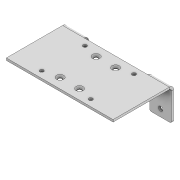
# Autodesk Inventor part: CCM_Mount_F
Saved by Autodesk Inventor 2020 (Build 240168000, 168)
## iProperties
Created: 2021-07-12
Part Number: CCM_Mount_F
Material: 一般
Document SubType Name: Sheet Metal
Designer: magnarecta
Density: 1 g/cm^3
Appearance: 既定
Sheet Metal Rule: Default
Author: magnarecta
Autodesk Inventor part; units mm, degrees
ref_plane "YZ Plane" through (0, 0, 0) normal (1, 0, 0) x (0, 1, 0)
ref_plane "XZ Plane" through (0, 0, 0) normal (0, 1, 0) x (-1, 0, 0)
ref_plane "XY Plane" through (0, 0, 0) normal (0, 0, 1) x (1, 0, 0)
sketch "スケッチ1" plane through (0, 0, 0) normal (0, 1, 0) x (-1, 0, 0)
  line L0 (-40, -39) -> (40, -39)
  line L1 (40, -39) -> (40, 39)
  line L2 (40, 39) -> (-40, 39)
  line L3 (-40, 39) -> (-40, -39)
  line L4 (-40, -39) -> (40, 39) construction
  line L5 (40, -39) -> (-40, 39) construction
  point P0 (0, 0)
  dimension "d0" = 80
  dimension "d1" = 78
  constraints: 12 end point, 2 midpoint, 2 parallel, 1 horizontal, 1 perpendicular
  measures "d0" distance of L0.start L0.end
  measures "d1" distance of L0.end L1.end
extrude "押し出し1" add sketch "スケッチ1" along normal blind 3
sketch "スケッチ2" plane through (0, 3, 0) normal (0, 1, 0) x (1, 0, 0)
  line L0 (34, 30) -> (-34, 30)
  line L1 (-34, 30) -> (-34, -30)
  line L2 (-34, -30) -> (34, -30)
  line L3 (34, -30) -> (34, 30)
  line L4 (34, 30) -> (-34, -30) construction
  line L5 (-34, 30) -> (34, -30) construction
  point P0 (0, 0)
  dimension "d4" = 68
  dimension "d5" = 60
  constraints: 12 end point, 2 midpoint, 2 parallel, 1 horizontal, 1 perpendicular
  measures "d4" distance of L2.end L1.end
  measures "d5" distance of L1.end L0.end
hole "穴1" at (-34, 3, 30) at (34, 3, 30) at (34, 3, -30) at (-34, 3, -30) direction (0, -1, 0) diameter 5.2 depth 8 tip angle 118
sketch "スケッチ3" plane through (0, 3, 0) normal (0, 1, 0) x (1, 0, 0)
  line L0 (13.5, 25) -> (-13.5, 25)
  line L1 (-13.5, 25) -> (-13.5, -25)
  line L2 (-13.5, -25) -> (13.5, -25)
  line L3 (13.5, -25) -> (13.5, 25)
  line L4 (13.5, 25) -> (-13.5, -25) construction
  line L5 (-13.5, 25) -> (13.5, -25) construction
  point P0 (0, 0)
  dimension "d13" = 27
  dimension "d14" = 50
  constraints: 12 end point, 4 coincident, 2 midpoint, 2 parallel, 1 horizontal, 1 perpendicular
  measures "d13" distance of L0.start L0.end
  measures "d14" distance of L0.end L1.end
hole "穴2" at (-13.5, 3, 25) at (13.5, 3, 25) at (13.5, 3, -25) at (-13.5, 3, -25) direction (0, -1, 0) diameter 5.3 depth 8 tip angle 118 countersink diameter 10 countersink angle 90
sketch "スケッチ5" plane through (0, 0, 0) normal (0, -1, 0) x (1, 0, 0)
  line L0 (74, 39) -> (-74, 39)
  line L1 (-74, 39) -> (-74, -39)
  line L2 (-74, -39) -> (74, -39)
  line L3 (74, -39) -> (74, 39)
  circle A0 centre (13.5, -25) radius 2.65 projected
  circle A1 centre (34, -30) radius 2.6 projected
  circle A2 centre (-34, 30) radius 2.6 projected
  circle A3 centre (34, 30) radius 2.6 projected
  circle A4 centre (-34, -30) radius 2.6 projected
  line L4 (-40, -39) -> (-40, 39) projected
  line L5 (40, -39) -> (-40, -39) projected
  line L6 (40, 39) -> (40, -39) projected
  line L7 (-40, 39) -> (40, 39) projected
  point P0 (0, 0)
  point P1 (-40, 39)
  dimension "d28" = 40
  dimension "d29" = 40
  constraints: 8 end point, 2 horizontal alignment, 2 parallel, 1 horizontal, 1 perpendicular
  measures "d28" distance from line of A1.centre L3
  measures "d29" distance from line of L1 A4.centre
extrude "押し出し3" add sketch "スケッチ5" against normal up to surface (3 mm away) contours L3 L2 L6 L0 | L4 L2 L1 L0
sketch "スケッチ6" plane through (0, 0, 0) normal (0, -1, 0) x (1, 0, 0)
  circle A0 centre (34, -30) radius 2.6 projected
  circle A1 centre (-34, 30) radius 2.6 projected
  circle A2 centre (34, 30) radius 2.6 projected
  circle A3 centre (-34, -30) radius 2.6 projected
  line L0 (-74, -39) -> (74, -39) projected
  line L1 (74, -39) -> (74, 39) projected
  line L2 (74, 39) -> (-74, 39) projected
  line L3 (-74, 39) -> (-74, -39) projected
  line L4 (74, -39) -> (44, -39)
  line L5 (44, -39) -> (44, -42)
  line L6 (44, -42) -> (74, -42)
  line L7 (74, -42) -> (74, -39)
  line L8 (-74, 39) -> (-74, -39) projected
  line L9 (-74, -39) -> (-44, -39)
  line L10 (-44, -39) -> (-44, -42)
  line L11 (-44, -42) -> (-74, -42)
  line L12 (-74, -42) -> (-74, -39)
  line L13 (44, -42) -> (-44, -42)
  line L14 (-44, -42) -> (-44, -39)
  line L15 (-44, -39) -> (44, -39)
  line L16 (44, -39) -> (44, -42)
  point P0 (0, 0)
  dimension "d33" = 30
  dimension "d34" = 30
  dimension "d49" = 3
  constraints: 24 end point, 6 parallel, 3 horizontal, 3 perpendicular, 1 horizontal alignment
  measures "d33" distance of L5.end L6.end
  measures "d34" distance of L10.end L11.end
  measures "d49" distance of L11.end L0.start
extrude "押し出し5" add sketch "スケッチ6" against normal up to surface (3 mm away) contours L0 L10 L11 L12 | L0 L7 L6 L5
sketch "スケッチ8" plane through (74, 0, -42) normal (0, 0, -1) x (-1, 0, 0)
  line L0 (30, 0) -> (0, 0)
  line L1 (0, 0) -> (0, -42)
  line L2 (0, -42) -> (30, -42)
  line L3 (30, -42) -> (30, 0)
  constraints: 6 end point, 1 horizontal, 1 perpendicular, 1 vertical
edge flange "フランジ2" height 45 angle 90 thickness 3 bend radius 3 thickness toward (0, 0, -1) relief tear relief width 3 relief depth 1.5 corner gap 3 corner form 0 edges at (59, 0, -42) (-59, 0, -42) wall of the first edge with corners at (44, 0, -42) (74, 0, -42) (74, -42, -42) (44, -42, -42)
bend "曲げ2"
corner "コーナー2"
sketch "スケッチ9" plane through (-44, -42, -45) normal (0, 0, -1) x (-1, 0, 0)
  line L0 (30, 39) -> (0, 39) projected
  line L1 (0, 0) -> (0, 39) projected
  line L2 (30, 0) -> (0, 0) projected
  line L3 (30, 39) -> (30, 0) projected
  line L4 (-88, 39) -> (-118, 39) projected
  line L5 (-118, 0) -> (-118, 39) projected
  line L6 (-88, 0) -> (-118, 0) projected
  line L7 (-88, 39) -> (-88, 0) projected
  point P0 (-44, 42)
  point P1 (15, 10)
  point P2 (-103, 10)
  dimension "d62" = 10
  dimension "d63" = 15
  dimension "d64" = 15
  constraints: 1 horizontal alignment
  measures "d62" distance from line of point (15, 10) L2
  measures "d63" distance from line of point (15, 10) L3
  measures "d64" distance from line of L5 point (-103, 10)
hole "穴3" at (-59, -32, -45) at (59, -32, -45) direction (0, 0, 1) diameter 6.2 depth 3 tip angle 118
fillet "フィレット3" radius 2 4 edges at (-74, -42, -43.5) (-44, -42, -43.5) (44, -42, -43.5) (74, -42, -43.5)
equation "\"d28\" = d29"
equation "\"d70\" = Thickness"
equation "\"d38\" = Thickness"
equation "\"d52\" = BendReliefWidth"
equation "\"d53\" = BendReliefDepth"
equation "\"d54\" = MinimumRemnant"
equation "\"d55\" = TransitionRadius"
equation "\"d58\" = BendRadius"
equation "\"d59\" = CornerReliefSize"
equation "\"d60\" = GapSize"
equation "\"d61\" = JacobiRadiusSize"
equation "\"BendRadius\" = Thickness"
equation "\"BendReliefWidth\" = Thickness"
equation "\"BendReliefDepth\" = 0.5 * Thickness"
equation "\"CornerReliefSize\" = 4 * Thickness"
equation "\"MinimumRemnant\" = 2 * Thickness"
equation "\"TransitionRadius\" = BendRadius"
equation "\"JacobiRadiusSize\" = Thickness"
equation "\"GapSize\" = Thickness"
equation "\"Thickness\" = 3"
